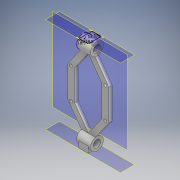
# Autodesk Inventor part: mousetrapMount
Saved by Autodesk Inventor 2018 (Build 220112000, 112)
## iProperties
Created: 2018-11-24
Part Number: mousetrapMount
Material: Generic
Document SubType Name: Modeling
Designer: Prakash
Density: 1 g/cm^3
Appearance: Default
Author: Prakash
Autodesk Inventor part; units mm, degrees
ref_plane "YZ Plane" through (0, 0, 0) normal (1, 0, 0) x (0, 1, 0)
ref_plane "XY Plane" through (0, 0, 0) normal (0, 0, 1) x (1, 0, 0)
sketch "Sketch3" plane through (0, 0, 0) normal (1, 0, 0) x (0, 1, 0)
  circle A0 centre (0, 0) radius 5.25
  circle A1 centre (0, 0) radius 9.25
  dimension "d0" = 10.5
  dimension "d1" = 18.5
  constraints: 2 centre point, 2 coincident
  measures "d0" diameter of A0
  measures "d1" diameter of A1
extrude "Extrusion1" add sketch "Sketch3" along normal blind 20
ref_plane "Work Plane1" through (0, 9.25, 0) normal (0, 1, 0) x (-1, 0, 0)
sketch "Sketch4" plane through (0, 9.25, 0) normal (0, 1, 0) x (-1, 0, 0)
  line L0 (-20, 9.25) -> (-20, -9.25) projected
  line L1 (-20, 0) -> (0, 0) construction
  line L2 (0, 9.25) -> (-20, 9.25) projected
  line L3 (-20, 9.25) -> (-20, -9.25) projected
  line L4 (0, -9.25) -> (0, 9.25) projected
  line L5 (0, -9.25) -> (-20, -9.25) construction
  line L6 (-59.213, -14.8) -> (39.213, -14.8) construction
  line L7 (39.213, -14.8) -> (39.213, -59.25) construction
  line L8 (39.213, -59.25) -> (-59.213, -59.25) construction
  line L9 (-59.213, -59.25) -> (-59.213, -14.8) construction
  line L10 (-59.213, -14.8) -> (39.213, -59.25) construction
  line L11 (39.213, -14.8) -> (-59.213, -59.25) construction
  line L12 (-59.213, -59.25) -> (39.213, -59.25) construction
  line L13 (39.213, -59.25) -> (39.213, -103.7) construction
  line L14 (39.213, -103.7) -> (-59.213, -103.7) construction
  line L15 (-59.213, -103.7) -> (-59.213, -59.25) construction
  line L16 (-59.213, -59.25) -> (39.213, -103.7) construction
  line L17 (39.213, -59.25) -> (-59.213, -103.7) construction
  line L18 (-10, -37.025) -> (-59.213, -37.025) construction
  line L19 (-10, -37.025) -> (39.213, -37.025) construction
  line L20 (-10, -81.475) -> (-59.213, -81.475) construction
  line L21 (-10, -81.475) -> (39.213, -81.475) construction
  line L22 (-20, -9.25) -> (-39.6065, -37.025)
  line L23 (-10, -9.25) -> (-29.6065, -37.025)
  line L24 (-39.6065, -37.025) -> (-39.6065, -59.25)
  line L25 (-10, -9.25) -> (9.6065, -37.025)
  line L26 (0, -9.25) -> (19.6065, -37.025)
  line L27 (19.6065, -37.025) -> (19.6065, -59.25)
  line L28 (-34.6065, -37.025) -> (-34.6065, -81.475) construction
  line L29 (14.6065, -81.475) -> (14.6065, -37.025) construction
  line L30 (-29.6065, -37.025) -> (-29.6065, -59.25)
  line L31 (9.6065, -37.025) -> (9.6065, -59.25)
  line L32 (-39.6065, -59.25) -> (-29.6065, -59.25)
  line L33 (9.6065, -59.25) -> (19.6065, -59.25)
  line L34 (-20, -9.25) -> (-10, -9.25)
  line L35 (0, -9.25) -> (-20, -9.25) projected
  line L36 (-10, -9.25) -> (0, -9.25)
  point P0 (-10, 0)
  dimension "d5" = 44.45
  dimension "d6" = 49.213
  dimension "d7" = 44.45
  dimension "d21" = 50
  constraints: 62 end point, 15 midpoint, 10 point on line, 8 parallel, 5 perpendicular, 3 horizontal, 2 collinear, 2 vertical, 1 equal length, 2 other
  measures "d5" distance of L6.end L7.end
  measures "d6" distance from line of L7 L18.start
  measures "d7" distance of L12.end L13.end
  measures "d21" distance between parallel lines of L8 L5
ref_plane "Work Plane2" through (0, 0, 0) normal (0, 1, 0) x (-1, 0, 0)
sketch "Sketch5" plane through (0, 0, 0) normal (0, 1, 0) x (-1, 0, 0)
  line L0 (-20, -9.25) -> (-39.6065, -37.025) projected
  line L1 (-10, -9.25) -> (-29.6065, -37.025) projected
  line L2 (-10, -9.25) -> (9.6065, -37.025) projected
  line L3 (0, -9.25) -> (19.6065, -37.025) projected
  line L4 (19.6065, -37.025) -> (19.6065, -59.25) projected
  line L5 (9.6065, -37.025) -> (9.6065, -59.25) projected
  line L6 (-29.6065, -37.025) -> (-29.6065, -59.25) projected
  line L7 (-39.6065, -37.025) -> (-39.6065, -59.25) projected
  line L8 (-39.6065, -59.25) -> (-29.6065, -59.25) projected
  line L9 (9.6065, -59.25) -> (19.6065, -59.25) projected
  line L10 (0, -9.25) -> (-20, -9.25) projected
  point P0 (0, 0)
  point P1 (-34.6065, -37.025)
  point P2 (14.6065, -37.025)
extrude "Extrusion2" add sketch "Sketch5" along normal mid plane 5
sketch "Sketch7" plane through (0, -2.5, 0) normal (0, -1, 0) x (1, 0, 0)
  point P0 (0, 0)
  point P1 (34.6065, -37.025)
  point P2 (-14.6065, -37.025)
hole "Hole1" at (-14.6065, -2.5, -37.025) at (34.6065, -2.5, -37.025) direction (0, 1, 0) diameter 4.305 end through all clearance for "Flat Head Machine Screw (82)" size "#6" standard "Ansi Unified Screw Threads"
sketch "Sketch8" plane through (0, 0, -9.25) normal (0, 0, 1) x (1, 0, 0)
  line L0 (0, 2.5) -> (10, 2.5) projected
  line L1 (20, 0) -> (20, -2.5) projected
  line L2 (0, 2.5) -> (20, 2.5)
  line L3 (20, 2.5) -> (20, -2.5)
  line L4 (20, -2.5) -> (0, -2.5)
  line L5 (0, -2.5) -> (0, 2.5)
  point P0 (0, 0)
  constraints: 8 end point, 2 parallel, 1 horizontal, 1 perpendicular
extrude "Extrusion4" add sketch "Sketch8" along normal up to surface round surface about axis through (0, 0, 0) along (1, 0, 0) radius 9.25 far side no
mirror "Mirror2" about plane through (-9.6065, 0, -59.25) normal (0, 0, -1) of "Extrusion1", "Extrusion2", "Hole1"
ref_plane "Work Plane3" through (0, 0, 9.25) normal (0, 0, -1) x (-1, 0, 0)
sketch "Sketch9" plane through (0, 0, 9.25) normal (0, 0, -1) x (-1, 0, 0)
  line L0 (0, 9.25) -> (-20, 9.25) projected
  line L1 (0, -9.25) -> (-20, -9.25) projected
  line L2 (-20, 9.25) -> (0, 9.25) projected
  line L3 (-3.3125, 9.25) -> (-3.3125, -9.25)
  line L4 (-3.3125, -9.25) -> (-16.6875, -9.25)
  line L5 (-20, -9.25) -> (0, -9.25) projected
  line L6 (-16.6875, 9.25) -> (-16.6875, -9.25)
  line L7 (-16.6875, 9.25) -> (-3.3125, 9.25)
  line L8 (-10, 9.25) -> (-10, -9.25) construction
  point P0 (0, 0)
  dimension "d24" = 13.3751
  constraints: 10 end point, 4 point on line, 3 perpendicular, 2 midpoint, 1 other
  measures "d24" distance between parallel lines of L6 L3
ref_plane "Work Plane4" through (0, 0, -127.75) normal (0, 0, -1) x (-1, 0, 0)
sketch "Sketch10" plane through (0, 0, -127.75) normal (0, 0, -1) x (-1, 0, 0)
  line L0 (-3.3125, 9.25) -> (-3.3125, -9.25) projected
  line L1 (0, 9.25) -> (-20, 9.25) projected
  line L2 (-16.6875, 9.25) -> (-16.6875, -9.25) projected
  line L3 (-10, 9.25) -> (-10, -9.25) construction
  line L4 (0, -9.25) -> (-20, -9.25) projected
  point P0 (0, 0)
extrude "Extrusion5" add sketch "Sketch10" against normal up to surface round surface about axis through (0, 0, -118.5) along (-1, 0, 0) radius 9.25 far side no
equation "\"d7\" = d5"
body "Solid1"
